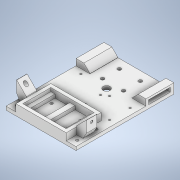
# Autodesk Inventor part: chassis
Saved by Autodesk Inventor 2022 (Build 260153000, 153)
## iProperties
Created: 2021-04-16
Part Number: chassis
Material: Plastic, Opaque White
Document SubType Name: Modeling
Designer: kevin
Density: 0.952 g/cm^3
Appearance: Smooth - White
Author: kevin
Autodesk Inventor part; units mm, degrees
ref_plane "YZ Plane" through (0, 0, 0) normal (1, 0, 0) x (0, 1, 0)
ref_plane "XZ Plane" through (0, 0, 0) normal (0, 1, 0) x (-1, 0, 0)
ref_plane "XY Plane" through (0, 0, 0) normal (0, 0, 1) x (1, 0, 0)
sketch "Sketch1" plane through (0, 0, 0) normal (0, 1, 0) x (-1, 0, 0)
  line L0 (63.5, 88.9) -> (-63.5, 88.9)
  line L1 (-63.5, 88.9) -> (-63.5, -88.9)
  line L2 (-63.5, -88.9) -> (63.5, -88.9)
  line L3 (63.5, -88.9) -> (63.5, 88.9)
  line L4 (63.5, 88.9) -> (-63.5, -88.9) construction
  line L5 (-63.5, 88.9) -> (63.5, -88.9) construction
  point P0 (0, 0)
  dimension "d0" = 177.8
  dimension "d1" = 127
  constraints: 12 end point, 2 midpoint, 2 parallel, 1 horizontal, 1 perpendicular
  measures "d0" distance of L2.end L0.start
  measures "d1" distance of L0.start L0.end
extrude "main chassis frame" add sketch "Sketch1" along normal blind 6.35
sketch "Sketch4" plane through (0, 6.35, 0) normal (0, 1, 0) x (1, 0, 0)
  circle A0 centre (54.8311, -78.0654) radius 2.3812
  circle A1 centre (54.8311, -43.3944) radius 2.3812
  line L0 (54.8311, -75.6842) -> (54.8311, -45.7757) construction
  circle A2 centre (26.4212, -78.0654) radius 2.3812
  circle A3 centre (26.4212, -43.3944) radius 2.3812
  line L1 (26.4212, -75.6842) -> (26.4212, -45.7757) construction
  line L2 (28.8024, -78.0654) -> (52.4498, -78.0654) construction
  point P0 (0, 0)
  dimension "d19" = 4.7625
  dimension "d165" = 4.7625
  dimension "d164" = 29.9085
  dimension "d166" = 29.9085
  dimension "d167" = 23.6474
  constraints: 6 end point, 4 point on circle, 2 centre point, 2 vertical, 2 vertical alignment, 1 horizontal, 6 other
  measures "d164" distance of L0.start L0.end
  measures "d166" distance of L1.start L1.end
  measures "d167" distance of L2.start L2.end
extrude "mounting holes for caster" cut sketch "Sketch4" against normal blind 6.35
sketch "Sketch5" plane through (0, 6.35, 0) normal (0, 1, 0) x (1, 0, 0)
  line L0 (63.5, 88.9) -> (-63.5, 88.9) projected
  line L1 (-63.5, -88.9) -> (63.5, -88.9) projected
  line L2 (0, 88.9) -> (-63.5, 88.9)
  line L3 (-63.5, 88.9) -> (-63.5, -88.9)
  line L4 (-63.5, -88.9) -> (0, -88.9)
  line L5 (0, -88.9) -> (0, 88.9)
  point P0 (0, 0)
  point P1 (-63.5, 88.9)
  constraints: 8 end point, 2 parallel, 1 horizontal, 1 midpoint, 1 perpendicular
extrude "cut in half to mirror holes later" cut sketch "Sketch5" against normal blind 6.35
sketch "Sketch6" plane through (0, 0, 0) normal (0, -1, 0) x (1, 0, 0)
  circle A0 centre (19.05, -72.3766) radius 3.175
  line L0 (63.5378, -72.3766) -> (19.0878, -72.3766) construction
  line L1 (19.0878, -72.3766) -> (19.0878, -41.8966) construction
  circle A1 centre (19.0878, -41.8966) radius 3.175
  point P0 (0, 0)
  dimension "d26" = 44.45
  dimension "d27" = 6.35
  dimension "d28" = 30.48
  dimension "d29" = 6.35
  constraints: 4 end point, 2 centre point, 1 coincident, 1 horizontal, 1 vertical
  measures "d26" distance of L0.start L0.end
  measures "d27" diameter of A0
  measures "d28" distance of L0.end L1.end
  measures "d29" diameter of A1
extrude "zip tie mounting holes for motors" cut sketch "Sketch6" against normal blind 6.35
sketch "Sketch12" plane through (0, 6.35, 0) normal (0, 1, 0) x (1, 0, 0)
  line L0 (63.5, 88.9) -> (0, 88.9) projected
  line L1 (63.5, 88.9) -> (38.1, 88.9)
  line L2 (38.1, 88.9) -> (38.1, 38.1)
  line L3 (38.1, 38.1) -> (63.5, 38.1)
  line L4 (63.5, 38.1) -> (63.5, 88.9)
  point P0 (0, 0)
  dimension "d227" = 50.8
  dimension "d228" = 25.4
  constraints: 8 end point, 2 parallel, 1 horizontal, 1 perpendicular
  measures "d227" distance of L1.end L2.end
  measures "d228" distance of L2.end L3.end
extrude "motor mount covers" add sketch "Sketch12" along normal blind 11.43
chamfer "motor mount slants" distance 11.1125 angle 45 1 edges at (38.1, 17.78, -63.5)
mirror "Mirror6" about plane through (0, 0, 0) normal (1, 0, 0)
sketch "Sketch22" plane through (0, 6.35, 0) normal (0, 1, 0) x (1, 0, 0)
  circle A0 centre (0, 30.1625) radius 6.35
  point P0 (0, 0)
  constraints: 1 centre point
extrude "new hole for motor wires" cut sketch "Sketch22" against normal blind 6.35
sketch "arduino uno mounting holes" plane through (0, 6.35, 0) normal (0, 1, 0) x (1, 0, 0)
  line L0 (-63.5, -88.9) -> (-63.5, 88.9) projected
  line L1 (-58.42, -17.7229) -> (-58.42, 33.0771) construction
  circle A0 centre (-46.0375, 29.5275) radius 1.778
  circle A1 centre (-47.3075, -18.7325) radius 1.778
  circle A2 centre (4.7625, 14.2875) radius 1.778
  circle A3 centre (4.7625, -13.6525) radius 1.778
  line L2 (-46.0375, 34.2699) -> (-46.0375, -23.7548) construction
  line L3 (-47.3075, -22.4854) -> (-47.3075, 33.7972) construction
  line L4 (4.7625, -21.8575) -> (4.7625, 22.1977) construction
  line L5 (15.8332, 14.2875) -> (-15.1882, 14.2875) construction
  line L6 (-52.07, 29.5275) -> (-2.2478, 29.5275) construction
  line L7 (11.43, -13.6525) -> (-14.3019, -13.6525) construction
  line L8 (-51.7639, -18.7325) -> (-2.8575, -18.7325) construction
  point P0 (0, 0)
  dimension "d186" = 3.556
  dimension "d219" = 1.27
  dimension "d220" = 15.24
  dimension "d221" = 27.94
  dimension "d222" = 5.08
  dimension "d223" = 50.8
  constraints: 16 end point, 8 point on line, 4 centre point, 3 equal radius, 3 horizontal, 3 vertical
  measures "d186" diameter of A2
  measures "d219" distance between parallel lines of L3 L2
  measures "d220" distance between parallel lines of L5 L6
  measures "d221" distance between parallel lines of L7 L5
  measures "d222" distance between parallel lines of L8 L7
  measures "d223" distance between parallel lines of L4 L2
extrude "uno mounting holes" cut sketch "arduino uno mounting holes" against normal blind 6.35
sketch "motor mount holes sketch" plane through (0, 6.35, 0) normal (0, 1, 0) x (1, 0, 0)
  line L0 (12.2391, 24.4663) -> (55.7366, 24.4663) construction
  line L1 (55.7366, 24.4663) -> (55.7366, -19.0312) construction
  line L2 (55.7366, -19.0312) -> (12.2391, -19.0312) construction
  line L3 (12.2391, -19.0312) -> (12.2391, 24.4663) construction
  circle A0 centre (52.0566, 20.7844) radius 1.778
  line L4 (52.1191, 22.5613) -> (52.1191, 24.4663) construction
  line L5 (53.8316, 20.8881) -> (55.7366, 20.8881) construction
  circle A1 centre (14.5948, 20.8847) radius 1.778
  line L6 (16.206, 21.6364) -> (50.496, 21.6364) construction
  circle A2 centre (52.1171, -16.6794) radius 1.778
  line L7 (52.888, -15.0773) -> (52.888, 19.2127) construction
  circle A3 centre (14.6521, -16.6794) radius 1.778
  line L8 (16.2396, -15.8787) -> (50.5296, -15.8787) construction
  point P0 (0, 0)
  dimension "d224" = 3.556
  dimension "d208" = 43.4975
  dimension "d209" = 43.4975
  dimension "d210" = 1.905
  dimension "d211" = 1.905
  dimension "d214" = 34.29
  dimension "d215" = 34.29
  dimension "d216" = 34.29
  constraints: 18 end point, 6 point on circle, 3 parallel, 3 perpendicular, 2 centre point, 2 horizontal, 2 point on line, 1 vertical, 12 other
  measures "d208" distance of L2.end L0.start
  measures "d209" distance of L0.start L0.end
  measures "d210" distance of L4.start L4.end
  measures "d211" distance of L5.start L5.end
  measures "d214" distance of L6.start L6.end
  measures "d215" distance of L7.start L7.end
  measures "d216" distance of L8.start L8.end
extrude "L298N mount holes" cut sketch "motor mount holes sketch" against normal blind 6.6675
sketch "Sketch33" plane through (0, 6.35, 0) normal (0, 1, 0) x (1, 0, 0)
  line L0 (-45.72, -25.4) -> (45.72, -25.4)
  line L1 (45.72, -25.4) -> (45.72, -88.9)
  line L2 (45.72, -88.9) -> (-45.72, -88.9)
  line L3 (-45.72, -88.9) -> (-45.72, -25.4)
  line L4 (-39.37, -31.75) -> (39.37, -31.75)
  line L5 (39.37, -31.75) -> (39.37, -82.55)
  line L6 (39.37, -82.55) -> (-39.37, -82.55)
  line L7 (-39.37, -82.55) -> (-39.37, -31.75)
  line L8 (-45.72, -60.325) -> (-63.5, -60.325) construction
  line L9 (-63.5, -88.9) -> (-63.5, 88.9) projected
  line L10 (45.72, -65.0875) -> (63.5, -65.0875) construction
  line L11 (63.5, -88.9) -> (63.5, 88.9) projected
  line L12 (-63.5, -88.9) -> (63.5, -88.9) projected
  point P0 (0, 0)
  dimension "d235" = 63.5
  dimension "d236" = 50.8
  dimension "d237" = 91.44
  dimension "d238" = 78.74
  dimension "d239" = 6.35
  dimension "d240" = 6.35
  dimension "d241" = 6.35
  dimension "d242" = 6.35
  constraints: 20 end point, 5 parallel, 4 horizontal, 4 point on line, 2 perpendicular, 1 collinear
  measures "d235" distance between parallel lines of L2 L0
  measures "d236" distance of L4.end L5.end
  measures "d237" distance between parallel lines of L3 L1
  measures "d238" distance between parallel lines of L5 L7
  measures "d239" distance between parallel lines of L4 L0
  measures "d240" distance between parallel lines of L2 L6
  measures "d241" distance between parallel lines of L3 L7
  measures "d242" distance between parallel lines of L5 L1
extrude "battery walls" add sketch "Sketch33" along normal blind 12.7
sketch "Sketch34" plane through (0, 6.35, 0) normal (0, 1, 0) x (1, 0, 0)
  line L0 (39.37, -31.75) -> (-39.37, -31.75) projected
  line L1 (-39.37, -82.55) -> (39.37, -82.55) projected
  line L2 (-31.75, -31.75) -> (-39.37, -31.75)
  line L3 (-39.37, -31.75) -> (-39.37, -82.55)
  line L4 (-39.37, -82.55) -> (-31.75, -82.55)
  line L5 (-31.75, -82.55) -> (-31.75, -31.75)
  line L6 (39.37, -82.55) -> (39.37, -31.75) projected
  line L7 (39.37, -31.75) -> (31.75, -31.75)
  line L8 (31.75, -31.75) -> (31.75, -82.55)
  line L9 (31.75, -82.55) -> (39.37, -82.55)
  line L10 (39.37, -82.55) -> (39.37, -31.75)
  line L11 (4.7625, -31.75) -> (-4.7625, -31.75)
  line L12 (-4.7625, -31.75) -> (-4.7625, -82.55)
  line L13 (-4.7625, -82.55) -> (4.7625, -82.55)
  line L14 (4.7625, -82.55) -> (4.7625, -31.75)
  point P0 (0, 0)
  constraints: 24 end point, 6 parallel, 4 point on line, 3 horizontal, 3 perpendicular
extrude "battery inner walls" add sketch "Sketch34" along normal blind 6.35 contours L6 L1 L8 L0 | L14 L1 L12 L0 | L5 L1 L3 L0
sketch "Sketch32" plane through (63.5, 0, 88.9) normal (1, 0, 0) x (0, 0, -1)
  line L0 (171.196, 6.35) -> (131.826, 6.35)
  line L1 (131.826, 6.35) -> (131.826, 13.97)
  line L2 (131.826, 13.97) -> (171.196, 13.97)
  line L3 (171.196, 13.97) -> (171.196, 6.35)
  line L4 (171.196, 10.16) -> (177.8, 10.16) construction
  line L5 (177.8, 0) -> (177.8, 17.78) projected
  line L6 (131.826, 9.8881) -> (127, 9.8881) construction
  line L7 (127, 6.35) -> (127, 17.78) projected
  line L8 (0, 6.35) -> (127, 6.35) projected
  point P0 (88.9, 0)
  dimension "d225" = 39.37
  dimension "d226" = 7.62
  dimension "d268" = 6.604
  constraints: 12 end point, 3 horizontal, 3 point on line, 2 parallel, 1 collinear, 1 midpoint, 1 perpendicular
  measures "d225" distance of L1.end L2.end
  measures "d226" distance of L0.end L1.end
  measures "d268" distance of L4.start L4.end
extrude "motor mount slot - R" cut sketch "Sketch32" against normal blind 12.7
sketch "Sketch36" plane through (0, 6.35, 0) normal (0, 1, 0) x (1, 0, 0)
  line L0 (45.72, -88.9) -> (45.72, -25.4) projected
  line L1 (63.5, -88.9) -> (63.5, 88.9) projected
  line L2 (45.72, -69.85) -> (63.5, -69.85)
  line L3 (63.5, -69.85) -> (63.5, -50.9759)
  line L4 (63.5, -50.9759) -> (45.72, -50.9759)
  line L5 (45.72, -50.9759) -> (45.72, -69.85)
  point P0 (0, 0)
  constraints: 8 end point, 2 parallel, 2 point on line, 1 horizontal, 1 perpendicular
extrude "side panel mount pillar" add sketch "Sketch36" along normal blind 31.75
chamfer "side panel mount pillar slant" distance 17.4625 angle 45 1 edges at (45.72, 38.1, 60.4129)
sketch "side panel mount hole" plane through (63.5, 0, 88.9) normal (1, 0, 0) x (0, 0, -1)
  circle A0 centre (28.4871, 31.0499) radius 2.3812
  line L0 (28.4871, 31.0499) -> (19.05, 31.0499) construction
  line L1 (19.05, 6.35) -> (19.05, 38.1) projected
  line L2 (28.4871, 31.0499) -> (37.9241, 31.0499) construction
  line L3 (37.9241, 6.35) -> (37.9241, 38.1) projected
  circle A1 centre (28.4871, 31.0499) radius 3.175
  point P0 (88.9, 0)
  dimension "d256" = 4.7625
  dimension "d257" = 6.35
  constraints: 4 end point, 3 point on line, 2 centre point, 1 coincident, 1 collinear, 1 horizontal
  measures "d256" diameter of A0
  measures "d257" diameter of A1
extrude "side panel mount pillar hole - R" cut sketch "side panel mount hole" against normal blind 14.2875 contours A0 | A1
extrude "side panel mount pillar hole rim - R" add sketch "side panel mount hole" against normal blind 1.016
sketch "Sketch38" plane through (45.72, 6.35, 69.85) normal (0, 0, 1) x (1, 0, 0)
  line L0 (17.78, 0) -> (17.78, 11.43) projected
  line L1 (17.78, 11.43) -> (11.43, 0)
  line L2 (17.78, 0) -> (5.08, 0) projected
  point P0 (-45.72, -6.35)
  constraints: 2 end point, 1 midpoint
extrude "side panel mount pillar wire passageway - R" cut sketch "Sketch38" against normal blind 19.6215
mirror "Mirror7" about plane through (0, 0, 0) normal (1, 0, 0) of "motor mount slot - R", "side panel mount pillar", "side panel mount pillar slant", "side panel mount pillar hole - R", "side panel mount pillar hole rim - R", "side panel mount pillar wire passageway - R"
sketch "side panel hole dimensions" plane through (63.5, 0, 88.9) normal (1, 0, 0) x (0, 0, -1)
  line L0 (0, 0) -> (0, 6.35) projected
  line L1 (19.05, 17.78) -> (19.05, 38.1) projected
  circle A0 centre (28.4871, 31.0499) radius 2.3812 projected
  line L2 (177.8, 0) -> (177.8, 17.78) projected
  point P0 (88.9, 0)
  dimension "d264" = 19.05
  dimension "d265" = 9.4371
  dimension "d266" = 28.4871
  dimension "d267" = 149.3129
  measures "d264" distance between parallel lines of L0 L1
  measures "d265" distance from line of L1 A0.centre
  measures "d266" distance from line of L0 A0.centre
  measures "d267" distance from line of L2 A0.centre
body "Solid1"
